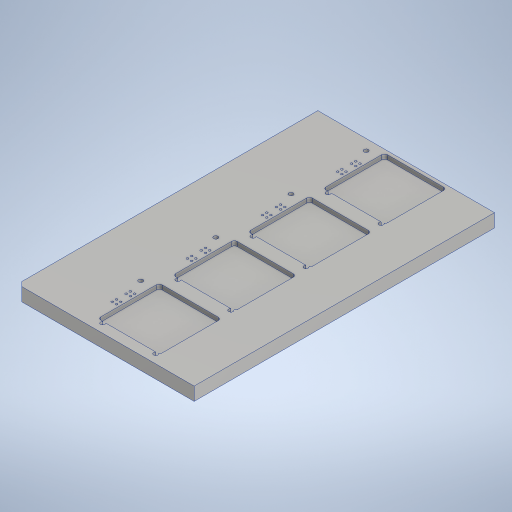
# Autodesk Inventor part: Assembly Plate
Saved by Autodesk Inventor 2023 (Build 270158000, 158)
## iProperties
Created: 2021-01-11
Part Number: Assembly Plate
Material: Aluminum 6061
Document SubType Name: Modeling
Designer: caleb
Density: 2.7 g/cm^3
Appearance: Aluminum - Flat
Author: caleb
Autodesk Inventor part; units mm, degrees
ref_plane "YZ Plane" through (0, 0, 0) normal (1, 0, 0) x (0, 1, 0)
ref_plane "XZ Plane" through (0, 0, 0) normal (0, 1, 0) x (-1, 0, 0)
ref_plane "XY Plane" through (0, 0, 0) normal (0, 0, 1) x (1, 0, 0)
sketch "Sketch1" plane through (0, 0, 0) normal (0, 1, 0) x (-1, 0, 0)
  line L0 (-63.5, 107.95) -> (63.5, 107.95)
  line L1 (63.5, 107.95) -> (63.5, -107.95)
  line L2 (63.5, -107.95) -> (-63.5, -107.95)
  line L3 (-63.5, -107.95) -> (-63.5, 107.95)
  line L4 (-63.5, 107.95) -> (63.5, -107.95) construction
  line L5 (63.5, 107.95) -> (-63.5, -107.95) construction
  point P0 (0, 0)
  dimension "d0" = 127
  dimension "d1" = 215.9
  constraints: 12 end point, 2 midpoint, 2 parallel, 1 horizontal, 1 perpendicular
  measures "d0" distance of L1.end L2.end
  measures "d1" distance of L0.end L1.end
extrude "Extrusion1" add sketch "Sketch1" along normal blind 9.525
chamfer "Chamfer1" distance 3.175 angle 45 1 edges at (-63.5, 4.7625, 107.95)
sketch "Sketch12" plane through (0, 9.525, 0) normal (0, 1, 0) x (1, 0, 0)
  circle A0 centre (-8.5, -101.6) radius 1.5875
  circle A1 centre (-21.2, -61.6) radius 1.5875
  circle A2 centre (29.6, -101.6) radius 1.5875
  line L0 (-63.5, 107.95) -> (-63.5, -104.775) projected
  line L1 (-60.325, -107.95) -> (63.5, -107.95) projected
  circle A3 centre (-21.2, -7.625) radius 1.5875
  circle A4 centre (-8.5, -47.625) radius 1.5875
  circle A5 centre (29.6, -47.625) radius 1.5875
  circle A6 centre (-21.2, 46.35) radius 1.5875
  circle A7 centre (-8.5, 6.35) radius 1.5875
  circle A8 centre (29.6, 6.35) radius 1.5875
  circle A9 centre (-21.2, 100.325) radius 1.5875
  circle A10 centre (-8.5, 60.325) radius 1.5875
  circle A11 centre (29.6, 60.325) radius 1.5875
  point P0 (0, 0)
  dimension "d166" = 3.175
  dimension "d167" = 38.1
  dimension "d169" = 12.7
  dimension "d170" = 40
  dimension "d196" = 53.975
  dimension "d254" = 55
  dimension "d255" = 6.35
  constraints: 12 centre point, 2 equal radius, 1 horizontal alignment, 1 vertical, 18 other
  measures "d166" diameter of A0
  measures "d167" distance of A2.centre A0.centre
  measures "d169" horizontal distance of A0.centre A1.centre
  measures "d170" vertical distance of A0.centre A1.centre
  measures "d196" distance of A1.centre A3.centre
  measures "d254" distance from line of L0 A0.centre
  measures "d255" distance from line of L1 A0.centre
extrude "Extrusion10" cut sketch "Sketch12" against normal through all
sketch "Sketch13" plane through (0, 9.525, 0) normal (0, 1, 0) x (1, 0, 0)
  line L0 (-60.325, -107.95) -> (63.5, -107.95) projected
  line L1 (-63.5, 107.95) -> (-63.5, -104.775) projected
  line L2 (-11.1125, -100.5125) -> (29.3875, -100.5125)
  line L3 (31.3875, -98.5125) -> (31.3875, -58.4125)
  line L4 (29.3875, -56.4125) -> (-11.1125, -56.4125)
  line L5 (-13.1125, -58.4125) -> (-13.1125, -98.5125)
  circle A0 centre (-21.2, -61.6) radius 1.5875 projected
  circle A1 centre (-8.5, -101.6) radius 1.5875 projected
  arc A2 (-13.1125, -98.5125) -> (-11.1125, -100.5125) centre (-11.1125, -98.5125) ccw
  arc A3 (-11.1125, -56.4125) -> (-13.1125, -58.4125) centre (-11.1125, -58.4125) ccw
  arc A4 (31.3875, -58.4125) -> (29.3875, -56.4125) centre (29.3875, -58.4125) ccw
  arc A5 (29.3875, -100.5125) -> (31.3875, -98.5125) centre (29.3875, -98.5125) ccw
  line L6 (-13.1125, -4.4375) -> (-13.1125, -44.5375)
  arc A6 (-13.1125, -44.5375) -> (-11.1125, -46.5375) centre (-11.1125, -44.5375) ccw
  line L7 (29.3875, -2.4375) -> (-11.1125, -2.4375)
  arc A7 (31.3875, -4.4375) -> (29.3875, -2.4375) centre (29.3875, -4.4375) ccw
  line L8 (31.3875, -44.5375) -> (31.3875, -4.4375)
  line L9 (-11.1125, -46.5375) -> (29.3875, -46.5375)
  arc A8 (29.3875, -46.5375) -> (31.3875, -44.5375) centre (29.3875, -44.5375) ccw
  arc A9 (-11.1125, -2.4375) -> (-13.1125, -4.4375) centre (-11.1125, -4.4375) ccw
  line L10 (-13.1125, 49.5375) -> (-13.1125, 9.4375)
  arc A10 (-13.1125, 9.4375) -> (-11.1125, 7.4375) centre (-11.1125, 9.4375) ccw
  line L11 (29.3875, 51.5375) -> (-11.1125, 51.5375)
  arc A11 (31.3875, 49.5375) -> (29.3875, 51.5375) centre (29.3875, 49.5375) ccw
  line L12 (31.3875, 9.4375) -> (31.3875, 49.5375)
  line L13 (-11.1125, 7.4375) -> (29.3875, 7.4375)
  arc A12 (29.3875, 7.4375) -> (31.3875, 9.4375) centre (29.3875, 9.4375) ccw
  arc A13 (-11.1125, 51.5375) -> (-13.1125, 49.5375) centre (-11.1125, 49.5375) ccw
  line L14 (-13.1125, 103.5125) -> (-13.1125, 63.4125)
  arc A14 (-13.1125, 63.4125) -> (-11.1125, 61.4125) centre (-11.1125, 63.4125) ccw
  line L15 (29.3875, 105.5125) -> (-11.1125, 105.5125)
  arc A15 (31.3875, 103.5125) -> (29.3875, 105.5125) centre (29.3875, 103.5125) ccw
  line L16 (31.3875, 63.4125) -> (31.3875, 103.5125)
  line L17 (-11.1125, 61.4125) -> (29.3875, 61.4125)
  arc A16 (29.3875, 61.4125) -> (31.3875, 63.4125) centre (29.3875, 63.4125) ccw
  arc A17 (-11.1125, 105.5125) -> (-13.1125, 103.5125) centre (-11.1125, 103.5125) ccw
  point P0 (0, 0)
  point P1 (-13.1125, -100.5125)
  point P2 (31.3875, -56.4125)
  point P3 (-13.1125, -56.4125)
  point P4 (-13.1125, -46.5375)
  point P5 (-13.1125, -2.4375)
  point P6 (31.3875, -2.4375)
  point P7 (-13.1125, 7.4375)
  point P8 (-13.1125, 51.5375)
  point P9 (31.3875, 51.5375)
  point P10 (-13.1125, 61.4125)
  point P11 (-13.1125, 105.5125)
  point P12 (31.3875, 105.5125)
  dimension "d241" = 44.5
  dimension "d242" = 44.1
  dimension "d243" = 2
  dimension "d246" = 53.975
  dimension "d252" = 1.0875
  dimension "d253" = 3.175
  dimension "d256" = 3.175
  dimension "d257" = 8.0875
  constraints: 32 end point, 32 point on circle, 24 point on line, 16 centre point, 8 tangent, 3 equal radius, 2 parallel, 1 horizontal, 1 perpendicular, 1 vertical, 69 other
  measures "d241" distance of point (31.387, -56.412) point (-13.113, -56.412)
  measures "d242" distance of point (-13.113, -56.412) point (-13.112, -100.512)
  measures "d243" radius of A2
  measures "d246" distance of point (-13.112, -100.512) point (-13.112, -46.537)
  measures "d252" distance from line of L2 A1.centre
  measures "d253" diameter of A1
  measures "d256" diameter of A0
  measures "d257" distance from line of L5 A0.centre
extrude "Extrusion11" cut sketch "Sketch13" against normal blind 3.175 contours A2 L5 A3 L4 A4 L3 A5 L2 A1 | A1 L2 | A9 L7 A7 L8 A8 L9 A6 L6 | A13 L11 A11 L12 A12 L13 A10 L10 | A17 L15 A15 L16 A16 L17 A14 L14 picked at (-8.5616, -100.3494)
sketch "Sketch14" plane through (0, 9.525, 0) normal (0, 1, 0) x (1, 0, 0)
  line L0 (-13.1125, -98.5125) -> (-13.1125, -58.4125) projected
  arc A0 (-9.6565, -100.5125) -> (-7.3435, -100.5125) centre (-8.5, -101.6) ccw projected
  point P0 (0, 0)
  point P1 (-18.3625, -84.9077)
  point P2 (-18.3625, -81.9077)
  point P3 (-15.3625, -81.9077)
  point P4 (-15.3625, -84.9077)
  point P5 (-18.3625, -74.9077)
  point P6 (-15.3625, -74.9077)
  point P7 (-18.3625, -71.9077)
  point P8 (-15.3625, -71.9077)
  point P9 (-15.3625, -17.9327)
  point P10 (-18.3625, -17.9327)
  point P11 (-15.3625, -20.9327)
  point P12 (-18.3625, -20.9327)
  point P13 (-15.3625, -30.9327)
  point P14 (-15.3625, -27.9327)
  point P15 (-18.3625, -27.9327)
  point P16 (-18.3625, -30.9327)
  point P17 (-15.3625, 36.0423)
  point P18 (-18.3625, 36.0423)
  point P19 (-15.3625, 33.0423)
  point P20 (-18.3625, 33.0423)
  point P21 (-15.3625, 23.0423)
  point P22 (-15.3625, 26.0423)
  point P23 (-18.3625, 26.0423)
  point P24 (-18.3625, 23.0423)
  point P25 (-15.3625, 90.0173)
  point P26 (-18.3625, 90.0173)
  point P27 (-15.3625, 87.0173)
  point P28 (-18.3625, 87.0173)
  point P29 (-15.3625, 77.0173)
  point P30 (-15.3625, 80.0173)
  point P31 (-18.3625, 80.0173)
  point P32 (-18.3625, 77.0173)
  dimension "d258" = 3
  dimension "d259" = 7
  dimension "d260" = 3
  dimension "d268" = 2.25
  dimension "d269" = 3
  dimension "d270" = 16.6923
  dimension "d273" = 53.975
  constraints: 5 vertical alignment, 4 horizontal alignment, 1 vertical, 24 other
  measures "d258" distance of point (-18.362, -81.908) point (-18.362, -84.908)
  measures "d259" distance of point (-18.362, -74.908) point (-18.362, -81.908)
  measures "d260" distance of point (-15.362, -84.908) point (-18.362, -84.908)
  measures "d268" distance from line of L0 point (-15.362, -84.908)
  measures "d269" distance of point (-18.362, -71.908) point (-18.362, -74.908)
  measures "d270" vertical distance of point (-18.362, -84.908) A0.centre
  measures "d273" distance of point (-15.362, -71.908) point (-15.363, -17.933)
hole "Hole3" at (-18.3625, 9.525, 84.9077) at (-18.3625, 9.525, 81.9077) at (-15.3625, 9.525, 81.9077) at (-15.3625, 9.525, 84.9077) at (-18.3625, 9.525, 74.9077) at (-15.3625, 9.525, 74.9077) at (-18.3625, 9.525, 71.9077) at (-15.3625, 9.525, 71.9077) at (-18.3625, 9.525, 30.9327) at (-18.3625, 9.525, 27.9327) at (-15.3625, 9.525, 27.9327) at (-15.3625, 9.525, 30.9327) at (-18.3625, 9.525, 20.9327) at (-15.3625, 9.525, 20.9327) at (-18.3625, 9.525, 17.9327) at (-15.3625, 9.525, 17.9327) at (-18.3625, 9.525, -77.0173) at (-18.3625, 9.525, -80.0173) at (-15.3625, 9.525, -80.0173) at (-15.3625, 9.525, -77.0173) at (-18.3625, 9.525, -87.0173) at (-15.3625, 9.525, -87.0173) at (-18.3625, 9.525, -90.0173) at (-15.3625, 9.525, -90.0173) at (-18.3625, 9.525, -23.0423) at (-18.3625, 9.525, -26.0423) at (-15.3625, 9.525, -26.0423) at (-15.3625, 9.525, -23.0423) at (-18.3625, 9.525, -33.0423) at (-15.3625, 9.525, -33.0423) at (-18.3625, 9.525, -36.0423) at (-15.3625, 9.525, -36.0423) direction (0, -1, 0) diameter 1.5 end through all
body "Solid1"
